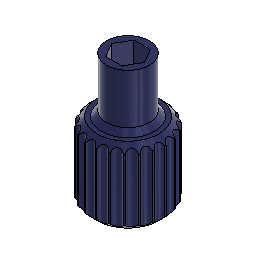
M8 nut adjuster (Autodesk Fusion 360 design; units mm, degrees)
Autodesk Fusion 360 part; units mm, degrees
sketch "Sketch1" plane through (0, 0, 0) normal (0, 0, 1) x (1, 0, 0)
  line L0 (2.396, -4.15) -> (4.792, 0)
  line L1 (4.792, 0) -> (2.396, 4.15)
  line L2 (2.396, 4.15) -> (-2.396, 4.15)
  line L3 (-2.396, 4.15) -> (-4.792, 0)
  line L4 (-4.792, 0) -> (-2.396, -4.15)
  line L5 (-2.396, -4.15) -> (2.396, -4.15)
  circle A0 centre (0, 0) radius 6.25
  circle A1 centre (0, 0) radius 11
  circle A2 centre (0, 11.5) radius 1.5
  line L6 (0, 11.5) -> (0, 0) construction
  dimension "d1" = 8.3
  dimension "d2" = 12.5
  dimension "d3" = 22
  dimension "d4" = 3
  dimension "d5" = 11.5
  constraint coincident A0.centre A1.centre
  constraint horizontal L2
  constraint vertical A0.centre A2.centre
  constraint coincident A2.centre L6.start
  measures "d1" distance of L2 L5
  measures "d2" diameter of A0
  measures "d3" diameter of A1
  measures "d4" diameter of A2
  measures "d5" distance of A2.centre A0.centre
extrude "Extrude1" add sketch "Sketch1" along normal blind 38 contours A0
extrude "Extrude2" add sketch "Sketch1" along normal blind 22 contours A1 A2 | A1 A2 picked at (-1.7308, 8.9775) picked at (0, 10.6602)
chamfer "Chamfer1" distance 2 angle 45 2 edges at (-10.2556, -3.9778, 0) (-10.2556, -3.9778, 22)
extrude "Extrude4" cut sketch "Sketch1" along normal through all contours A1 A2 picked at (0, 10.6602)
pattern_circular "C-Pattern1" count 22 over 360 about axis through (0, 0, 20) along (0, 0, 1) of "Extrude4"
chamfer "Chamfer2" distance 1.5 angle 45 1 edges at (-5.827, -2.2601, 22)
